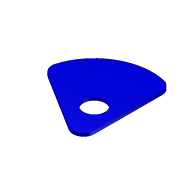
# Autodesk Inventor part: OpenROV 2_3 Dev EndCap Wire Guide Cover
Saved by Autodesk Inventor 2012 (Build 160160000, 160)
## iProperties
Created: 2011-09-29
Part Number: OpenROV 2_3 Dev EndCap Wire Guide Cover
Document SubType Name: Modeling
Designer: user
Density: 1 g/cm^3
Material: Default
Author: user
Autodesk Inventor part; units mm, degrees
ref_plane "YZ Plane" through (0, 0, 0) normal (1, 0, 0) x (0, 1, 0)
ref_plane "XZ Plane" through (0, 0, 0) normal (0, 1, 0) x (-1, 0, 0)
ref_plane "XY Plane" through (0, 0, 0) normal (0, 0, 1) x (1, 0, 0)
sketch "Sketch1" plane through (0, 0, 0) normal (0, 0, 1) x (1, 0, 0)
  line L0 (-47.415, 4.2576) -> (4.7008, -28.308)
  arc A0 (12.2727, 52.5869) -> (-51.6876, 15.6331) centre (0, 0) ccw
  line L1 (20, -19.8275) -> (20, 42.8486)
  arc A1 (-51.6876, 15.6331) -> (-47.415, 4.2576) centre (-42.1158, 12.7381) ccw
  arc A2 (20, 42.8486) -> (12.2727, 52.5869) centre (10, 42.8486) ccw
  arc A3 (4.7008, -28.308) -> (20, -19.8275) centre (10, -19.8275) ccw
  circle A4 centre (0, 0) radius 10
  point P0 (20, 50.1597)
  point P1 (-53.4041, 8)
  point P2 (20, 50.1597)
  point P3 (20, -37.868)
  point P4 (-53.4041, 8)
  dimension "d21" = 8
  dimension "d25" = 54
  dimension "d28" = 58
  dimension "d30" = 20
  dimension "d33" = 21.5155
  dimension "d38" = 10
  constraints: 11 point on circle, 6 point on line, 6 tangent, 5 centre point, 4 coincident, 4 end point, 2 equal radius
  measures "d21" vertical distance of point (0, 0) point (-53.404, 8)
  measures "d25" radius of A0
  measures "d28" angle of L1 L0
  measures "d30" distance from line of point (0, 0) L1
  measures "d33" distance from line of point (0, 0) L0
  measures "d38" radius of A1
extrude "Extrusion5" add sketch "Sketch1" along normal blind 3
body "Solid5"
